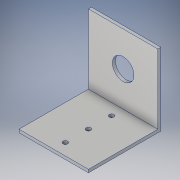
# Autodesk Inventor part: nhk14
Saved by Autodesk Inventor 2019 (Build 230136000, 136)
## iProperties
Created: 2022-02-15
Part Number: nhk14
Material: アルミニウム 6061
Document SubType Name: Sheet Metal
Designer: yuta
Density: 2.7 g/cm^3
Sheet Metal Rule: Default_mm
Appearance: アルミニウム - フラット
Author: yuta
Autodesk Inventor part; units mm, degrees
ref_plane "YZ Plane" through (0, 0, 0) normal (1, 0, 0) x (0, 1, 0)
ref_plane "XZ Plane" through (0, 0, 0) normal (0, 1, 0) x (-1, 0, 0)
ref_plane "XY Plane" through (0, 0, 0) normal (0, 0, 1) x (1, 0, 0)
sketch "スケッチ1" plane through (0, 0, 0) normal (0, 0, 1) x (1, 0, 0)
  line L0 (-12.8546, 6.7314) -> (32.1454, 6.7314)
  line L1 (32.1454, 6.7314) -> (32.1454, -38.2686)
  line L2 (32.1454, -38.2686) -> (-12.8546, -38.2686)
  line L3 (-12.8546, -38.2686) -> (-12.8546, 6.7314)
  point P0 (0, 0)
  dimension "d0" = 45
  dimension "d1" = 45
  constraints: 8 end point, 2 parallel, 1 horizontal, 1 perpendicular
  measures "d0" distance of L1.end L2.end
  measures "d1" distance of L0.end L1.end
sketch "スケッチ2" plane through (0, 0, 0) normal (0, 0, 1) x (1, 0, 0)
  point P0 (0, 0)
extrude "押し出し1" add sketch "スケッチ1" along normal blind 2
sketch "スケッチ3" plane through (0, 0, 2) normal (0, 0, 1) x (1, 0, 0)
  circle A0 centre (9.6454, -15.7686) radius 4
  line L0 (-12.8546, 6.7314) -> (-12.8546, -38.2686) projected
  line L1 (32.1454, 6.7314) -> (-12.8546, 6.7314) projected
  point P0 (0, 0)
  dimension "d4" = 8
  dimension "d5" = 22.5
  dimension "d6" = 45
  dimension "d7" = 22.5
  constraints: 1 centre point
  measures "d4" diameter of A0
  measures "d5" distance from line of L0 A0.centre
  measures "d6" distance of L0.start L0.end
  measures "d7" distance from line of L1 A0.centre
hole "穴1" at (9.6454, -15.7686, 2) direction (0, 0, -1) diameter 8 depth 2
sketch "スケッチ4" plane through (-12.8546, -38.2686, 0) normal (0, -1, 0) x (1, 0, 0)
  line L0 (0, 47) -> (45, 47)
  line L1 (45, 47) -> (45, 0)
  line L2 (45, 0) -> (0, 0)
  line L3 (0, 0) -> (0, 47)
  point P0 (12.8546, 0)
  dimension "d15" = 45
  dimension "d16" = 47
  constraints: 8 end point, 2 parallel, 1 coincident, 1 horizontal, 1 perpendicular
  measures "d15" distance of L1.end L2.end
  measures "d16" distance of L0.end L1.end
extrude "押し出し2" add sketch "スケッチ4" along normal blind 2
sketch "スケッチ5" plane through (0, 0, 2) normal (0, 0, 1) x (1, 0, 0)
  circle A0 centre (9.6454, -15.7686) radius 7
  line L0 (32.1454, 6.7314) -> (-12.8546, 6.7314) projected
  line L1 (32.1454, -38.2686) -> (32.1454, 6.7314) projected
  point P0 (0, 0)
  dimension "d19" = 14
  dimension "d20" = 22.5
  dimension "d21" = 22.5
  constraints: 1 centre point
  measures "d19" diameter of A0
  measures "d20" distance from line of L0 A0.centre
  measures "d21" distance from line of L1 A0.centre
extrude "押し出し3" cut sketch "スケッチ5" against normal blind 2
sketch "スケッチ6" plane through (-12.8546, -38.2686, 0) normal (0, 1, 0) x (1, 0, 0)
  circle A0 centre (22.5, -9.5) radius 1.5
  circle A1 centre (22.5, -24.5) radius 1.5
  circle A2 centre (22.5, -39.5) radius 1.5
  line L0 (45, -47) -> (45, -2) projected
  line L1 (0, -47) -> (45, -47) projected
  point P0 (12.8546, 0)
  dimension "d24" = 3
  dimension "d25" = 3
  dimension "d26" = 3
  dimension "d27" = 22.5
  dimension "d28" = 22.5
  dimension "d29" = 22.5
  dimension "d30" = 7.5
  dimension "d31" = 15
  dimension "d32" = 15
  constraints: 3 centre point
  measures "d24" diameter of A0
  measures "d25" diameter of A1
  measures "d26" diameter of A2
  measures "d27" distance from line of L0 A0.centre
  measures "d28" distance from line of L0 A1.centre
  measures "d29" distance from line of L0 A2.centre
  measures "d30" distance from line of L1 A2.centre
  measures "d31" distance of A2.centre A1.centre
  measures "d32" distance of A1.centre A0.centre
hole "穴2" at (9.6454, -38.2686, 39.5) at (9.6454, -38.2686, 24.5) at (9.6454, -38.2686, 9.5) direction (0, -1, 0) diameter 3 depth 2
equation "\"BendRadius\" = Thickness"
equation "\"BendReliefWidth\" = Thickness"
equation "\"BendReliefDepth\" = 0.5 * Thickness"
equation "\"CornerReliefSize\" = 4 * Thickness"
equation "\"MinimumRemnant\" = 2 * Thickness"
equation "\"TransitionRadius\" = BendRadius"
equation "\"JacobiRadiusSize\" = BendRadius"
equation "\"GapSize\" = Thickness"
equation "\"Thickness\" = 0.5"
